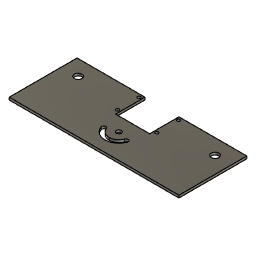
HeadMounter (Autodesk Fusion 360 design; units mm, degrees)
Autodesk Fusion 360 part; units mm, degrees
sketch "Sketch1" plane through (0, 0, 0) normal (0, 0, 1) x (1, 0, 0)
  line L0 (-86.36, 75.6587) -> (53.34, 75.6587)
  line L1 (53.34, 75.6587) -> (53.34, 19.7787)
  line L2 (53.34, 19.7787) -> (-86.36, 19.7787)
  line L3 (-86.36, 19.7787) -> (-86.36, 75.6587)
  circle A0 centre (-72.8218, 63.0603) radius 3.175
  circle A1 centre (39.8018, 63.0603) radius 3.175
  line L4 (-30.5054, 75.6587) -> (-2.5146, 75.6587)
  line L5 (-2.5146, 75.6587) -> (-2.5146, 51.5287)
  line L6 (-2.5146, 51.5287) -> (-30.5054, 51.5287)
  line L7 (-30.5054, 51.5287) -> (-30.5054, 75.6587)
  circle A2 centre (-32.7914, 73.0679) radius 1.27
  circle A3 centre (-32.7914, 55.3387) radius 1.27
  circle A4 centre (-0.2286, 73.0679) radius 1.27
  circle A5 centre (-0.2286, 55.2371) radius 1.27
  circle A6 centre (-16.51, 40.2003) radius 2.0574
  line L8 (-16.51, 50.9873) -> (-16.51, 22.86) construction
  circle A7 centre (-25.7048, 36.9237) radius 1.7272
  circle A8 centre (-16.51, 30.4467) radius 1.7272 construction
  circle A9 centre (-7.3152, 36.9237) radius 1.7272
  line L9 (-25.7048, 36.9237) -> (-7.3152, 36.9237) construction
  line L10 (-24.7101, 38.3357) -> (-15.5153, 31.8587) construction
  line L11 (-17.721, 31.6783) -> (-8.3127, 38.3337) construction
  line L12 (-17.5047, 29.0346) -> (-26.6995, 35.5116) construction
  line L13 (-15.5153, 29.0346) -> (-6.3205, 35.5116) construction
  circle A10 centre (-16.51, 40.2003) radius 9.7612 construction
  circle A11 centre (-16.51, 40.2003) radius 11.4884 construction
  arc A12 (-27.3318, 36.3439) -> (-16.51, 28.7195) centre (-16.5207, 40.1964) ccw
  arc A13 (-16.51, 28.7195) -> (-5.6882, 36.3439) centre (-16.4993, 40.1964) ccw
  circle A14 centre (-16.5207, 40.1964) radius 8.0226 construction
  arc A15 (-24.0773, 37.5019) -> (-16.5119, 32.1739) centre (-16.5207, 40.1964) ccw
  arc A16 (-16.5119, 32.1739) -> (-8.9375, 37.5166) centre (-16.5208, 40.227) ccw
  dimension "d1" = 139.7
  dimension "d2" = 55.88
  dimension "d3" = 6.35
  dimension "d4" = 12.5984
  dimension "d5" = 13.5382
  dimension "d6" = 6.35
  dimension "d7" = 13.5382
  dimension "d9" = 27.9908
  dimension "d10" = 24.13
  dimension "d11" = 2.54
  dimension "d12" = 2.5908
  dimension "d13" = 2.286
  dimension "d14" = 2.5908
  dimension "d15" = 2.286
  dimension "d16" = 2.286
  dimension "d17" = 2.286
  dimension "d18" = 17.8308
  dimension "d19" = 17.7292
  dimension "d20" = 4.1148
  dimension "d23" = 11.3284
  dimension "d24" = 3.4544
  dimension "d25" = 3.4544
  dimension "d26" = 3.4544
  dimension "d27" = 18.3896
  dimension "d28" = 14.605
  dimension "d29" = 9.7536
  dimension "d30" = 12.5984
  constraint horizontal L0
  constraint vertical L1
  constraint horizontal L2
  constraint vertical L3
  constraint horizontal L4
  constraint vertical L5
  constraint horizontal L6
  constraint vertical L7
  constraint midpoint L0 L4
  constraint equal A2 A4
  constraint equal A2 A3
  constraint equal A4 A5
  constraint perpendicular L6 L8
  constraint coincident A6.centre L8
  constraint coincident L8 A8.centre
  constraint coincident A7.centre L9.start
  constraint coincident A9.centre L9.end
  constraint perpendicular L8 L9
  constraint midpoint L8 L9
  constraint coincident A7 L10.start
  constraint coincident A8 L10.end
  constraint tangent A8 L10
  constraint tangent A7 L10
  constraint coincident A8 L11.start
  constraint coincident A9 L11.end
  constraint tangent A9 L11
  constraint coincident A8 L12.start
  constraint coincident A7 L12.end
  constraint tangent A7 L12
  constraint tangent A8 L12
  constraint coincident A8 L13.start
  constraint coincident A9 L13.end
  constraint tangent A9 L13
  constraint tangent A8 L13
  constraint concentric A6 A10
  constraint coincident A9.centre A10
  constraint concentric A10 A11
  constraint tangent A7 A11
  constraint tangent A7 A12
  constraint coincident A7 A12.start
  constraint coincident A11 A12.start
  constraint coincident A8 A12.end
  constraint coincident L8 A12.end
  constraint tangent A9 A13
  constraint coincident A9 A13.end
  constraint coincident A11 A13.end
  constraint concentric A12 A14
  constraint tangent A8 A14
  constraint tangent A8 A15
  constraint coincident A14 A15.end
  constraint coincident A8 A15.end
  constraint coincident A14 A15.start
  constraint coincident A7 A15.start
  constraint tangent A14 A16
  constraint coincident A9 A16.end
  measures "d1" distance of L0.start L0.end
  measures "d2" distance of L0.start L2.end
  measures "d3" diameter of A0
  measures "d4" distance of L0 A0.centre
  measures "d5" distance of L3 A0.centre
  measures "d6" diameter of A1
  measures "d7" distance of L1 A1.centre
  measures "d9" distance of L4.start L4.end
  measures "d10" distance of L4.start L6.end
  measures "d11" diameter of A2
  measures "d12" distance of L0 A2.centre
  measures "d13" distance of L7 A2.centre
  measures "d14" distance of L0 A4.centre
  measures "d15" distance of L5 A4.centre
  measures "d16" distance of L5 A5.centre
  measures "d17" distance of L7 A3.centre
  measures "d18" distance of A4.centre A5.centre
  measures "d19" distance of A2.centre A3.centre
  measures "d20" diameter of A6
  measures "d23" distance of L6 A6.centre
  measures "d24" diameter of A7
  measures "d25" diameter of A8
  measures "d26" diameter of A9
  measures "d27" distance of A7.centre A9.centre
  measures "d28" distance of L6 A7.centre
  measures "d29" distance of A6.centre A8.centre
  measures "d30" distance of L0 A1.centre
extrude "Extrude1" add sketch "Sketch1" along normal blind 2.0066 contours L0 L1 L2 L3 L5 L6 L7
equation "d4 = ( 0.25 / 2 ) * 1 in + 0.371 in"
equation "d5 = ( 0.25 / 2 ) * 1 in + 0.408 in"
equation "d12 = ( 0.04 / 2 ) * 1 in + 0.082 in"
equation "d14 = ( 0.04 / 2 ) * 1 in + 0.082 in"
equation "d18 = 0.612 in + 0.09 in"
equation "d23 = 0.365 in + ( 0.162 / 2 ) * 1 in"
equation "d28 = 0.507 in + ( 0.136 / 2 ) * 1 in"
equation "d30 = d4"
